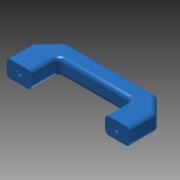
# Autodesk Inventor part: FrameHandle
Saved by Autodesk Inventor 2015 SP1 (Build 190203100, 203)
## iProperties
Created: 2015-04-26
Part Number: FrameHandle
Material: ABS Plastic
Document SubType Name: Modeling
Designer: Jack
Density: 1.06 g/cm^3
Appearance: Cyan
Author: Jack
Autodesk Inventor part; units mm, degrees
ref_plane "YZ Plane" through (0, 0, 0) normal (1, 0, 0) x (0, 1, 0)
ref_plane "XZ Plane" through (0, 0, 0) normal (0, 1, 0) x (-1, 0, 0)
ref_plane "XY Plane" through (0, 0, 0) normal (0, 0, 1) x (1, 0, 0)
sketch "Sketch1" plane through (0, 0, 0) normal (0, 0, 1) x (1, 0, 0)
  line L0 (0, 0) -> (0, 52)
  line L1 (0, 52) -> (148, 52)
  line L2 (148, 52) -> (148, 0)
  line L3 (148, 0) -> (118, 0)
  line L4 (118, 0) -> (118, 32)
  line L5 (118, 32) -> (30, 32)
  line L6 (30, 32) -> (30, 0)
  line L7 (30, 0) -> (0, 0)
  dimension "d0" = 52
  dimension "d1" = 88
  dimension "d2" = 30
  dimension "d3" = 32
  constraints: 16 end point, 7 perpendicular, 1 collinear, 1 point on line, 1 vertical
  measures "d0" distance of L0.start L0.end
  measures "d1" distance between parallel lines of L4 L6
  measures "d2" distance of L2.end L3.end
  measures "d3" distance of L5.end L6.end
extrude "Extrusion1" add sketch "Sketch1" along normal blind 20
chamfer "Chamfer1" distance 20 angle 45 2 edges at (0, 52, 10) (148, 52, 10)
fillet "Fillet1" radius 5 8 edges at (74, 32, 20) (30, 16, 20) (118, 16, 20) (74, 32, 0) (118, 16, 0) (30, 16, 0) (30, 32, 10) (118, 32, 10)
fillet "Fillet2" radius 5 10 edges at (0, 16, 20) (10, 42, 20) (74, 52, 20) (138, 42, 20) (148, 16, 20) (10, 42, 0) (0, 16, 0) (74, 52, 0) (138, 42, 0) (148, 16, 0)
fillet "Fillet3" radius 5 12 edges at (1.4645, 31.3934, 18.5355) (1.4645, 31.3934, 1.4645) (0, 32, 10) (20.6066, 50.5355, 1.4645) (20.6066, 50.5355, 18.5355) (20, 52, 10) (127.3934, 50.5355, 18.5355) (127.3934, 50.5355, 1.4645) (128, 52, 10) (146.5355, 31.3934, 1.4645) (146.5355, 31.3934, 18.5355) (148, 32, 10)
sketch "Sketch2" plane through (22.0711, 52, 5) normal (0, 1, 0) x (1, 0, 0)
  line L0 (-3.5355, 0) -> (-3.5355, -10) projected
  line L1 (-20.6066, 0) -> (-3.5355, 0) projected
  line L2 (-20.6066, -10) -> (-20.6066, 0) projected
  line L3 (-3.5355, -10) -> (-20.6066, -10) projected
  ellipse E0 centre (0, 0) end of major axis (0, -5) minor radius 3.5355 (0, 5) -> (-3.5355, 0) ccw projected
  line L4 (0, 5) -> (-17.0711, 5) projected
  ellipse E1 centre (-17.0711, 0) end of major axis (-17.0711, 5) minor radius 3.5355 (-17.0711, 5) -> (-20.6066, 0) ccw projected
  line L5 (-20.6066, 0) -> (-3.5355, 0) projected
  ellipse E2 centre (0, -10) end of major axis (0, -15) minor radius 3.5355 (-3.5355, -10) -> (0, -15) ccw projected
  line L6 (-3.5355, -10) -> (-20.6066, -10) projected
  ellipse E3 centre (-17.0711, -10) end of major axis (-17.0711, -5) minor radius 3.5355 (-20.6066, -10) -> (-17.0711, -15) ccw projected
  line L7 (-17.0711, -15) -> (0, -15) projected
  ellipse E4 centre (120.9289, 0) end of major axis (120.9289, -5) minor radius 3.5355 (124.4645, 0) -> (120.9289, 5) ccw projected
  line L8 (120.9289, 5) -> (103.8579, 5) projected
  ellipse E5 centre (103.8579, 0) end of major axis (103.8579, 5) minor radius 3.5355 (107.3934, 0) -> (103.8579, 5) ccw projected
  line L9 (107.3934, 0) -> (124.4645, 0) projected
  line L10 (124.4645, 0) -> (124.4645, -10) projected
  line L11 (107.3934, 0) -> (124.4645, 0) projected
  line L12 (107.3934, -10) -> (107.3934, 0) projected
  line L13 (124.4645, -10) -> (107.3934, -10) projected
  ellipse E6 centre (120.9289, -10) end of major axis (120.9289, -15) minor radius 3.5355 (120.9289, -15) -> (124.4645, -10) ccw projected
  line L14 (124.4645, -10) -> (107.3934, -10) projected
  ellipse E7 centre (103.8579, -10) end of major axis (103.8579, -5) minor radius 3.5355 (103.8579, -15) -> (107.3934, -10) ccw projected
  line L15 (103.8579, -15) -> (120.9289, -15) projected
  line L16 (-22.0711, 0) -> (-22.0711, -10) projected
  point P0 (-22.0711, 5)
  point P1 (-7.0711, -5)
  point P2 (109.4645, -5)
  dimension "d12" = 10
  dimension "d13" = 15
  dimension "d14" = 15
  constraints: 1 horizontal alignment, 8 other
  measures "d12" distance from line of L8 point (109.464, -5)
  measures "d13" distance from line of L16 point (-7.071, -5)
  measures "d14" distance from line of L10 point (109.464, -5)
hole "Hole1" at (15, 52, 10) at (131.5355, 52, 10) direction (0, -1, 0) diameter 5.2 end through all counterbore diameter 9 counterbore depth 37
chamfer "Chamfer2" distance 0.5 angle 45 6 edges at (10.9517, 42.9517, 8.035) (16.965, 48.965, 14.0483) (19.5, 51.2883, 10) (130.4697, 49.5303, 14.3719) (135.9075, 44.0925, 8.9341) (127.0355, 51.876, 10.0009)
body "Solid1"
